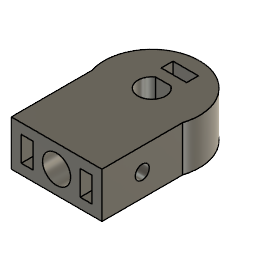
Union_encoder_péndulo (Autodesk Fusion 360 design; units mm, degrees)
Autodesk Fusion 360 part; units mm, degrees
sketch "Sketch1" plane through (0, 0, 0) normal (0, 0, 1) x (1, 0, 0)
  circle A0 centre (0, 0) radius 3.05
  circle A1 centre (0, 0) radius 10.5
  line L0 (-0.015271, 2.53) -> (-0.015271, 6.18)
  line L1 (-0.021322, 3.050767) -> (2.691698, 4.610144)
  line L2 (2.691698, 4.610144) -> (2.697749, 7.739376)
  line L3 (2.697749, 7.739376) -> (-0.009221, 9.309233)
  line L4 (-0.009221, 9.309233) -> (-2.722241, 7.749856)
  line L5 (-2.722241, 7.749856) -> (-2.728292, 4.620624)
  line L6 (-2.728292, 4.620624) -> (-0.021322, 3.050767)
  line L7 (-0.015271, 2.53) -> (1.703408, 2.53)
  line L8 (-0.015271, 2.53) -> (-1.703408, 2.53)
  point P0 (-0.015271, 6.18)
  dimension "d1" = 6.1
  dimension "d3" = 21
  dimension "d14" = 3.65
  dimension "d15" = 2.71
  constraint coincident A0.centre A1.centre
  constraint perpendicular L0 L7
  constraint perpendicular L0 L8
  measures "d1" diameter of A0
  measures "d3" diameter of A1
extrude "Extrude2" add sketch "Sketch1" along normal blind 8 contours L1 L2 L3 L4 L5 L6 | A0 L0 L7 | A0 L0 L8 | A1 picked at (-0.919611, 5.660208) picked at (0.132593, 2.866279) picked at (-0.165511, 2.864986) picked at (-5.003269, 3.445026)
sketch "Sketch3" plane through (0, 0, 8) normal (0, 0, 1) x (-1, 0, 0)
  circle A0 centre (0, 0) radius 10.5
  line L0 (0, 0) -> (0, -2.58)
  line L1 (0, -2.58) -> (0, -6.18)
  line L2 (-2.714531, -4.623256) -> (-2.705446, -7.752481)
  line L3 (-2.705446, -7.752481) -> (0.009086, -9.309225)
  line L4 (0.009086, -9.309225) -> (2.714531, -7.736744)
  line L5 (2.714531, -7.736744) -> (2.705446, -4.607519)
  line L6 (2.705446, -4.607519) -> (-0.009086, -3.050775)
  line L7 (-0.009086, -3.050775) -> (-2.714531, -4.623256)
  line L8 (2.75, -4.88) -> (-2.75, -4.88)
  line L9 (-2.75, -4.88) -> (-2.75, -7.48)
  line L10 (-2.75, -7.48) -> (2.75, -7.48)
  line L11 (2.75, -7.48) -> (2.75, -4.88)
  line L12 (2.75, -4.88) -> (-2.75, -7.48) construction
  line L13 (-2.75, -4.88) -> (2.75, -7.48) construction
  line L14 (1.703408, -2.53) -> (-1.703408, -2.53)
  arc A1 (1.703408, -2.53) -> (-1.703408, -2.53) centre (0, 0) ccw
  point P0 (0, -6.18)
  point P1 (0, -6.18)
  dimension "d18" = 2.58
  dimension "d19" = 3.6
  dimension "d20" = 2.71
  dimension "d36" = 5.5
  dimension "d37" = 2.6
  constraint coincident A0.centre L0.start
  constraint vertical L0
  constraint parallel L0 L1
  constraint coincident P1 P0
  constraint horizontal L8
  constraint perpendicular L8 L9
  constraint parallel L8 L10
  constraint parallel L9 L11
  constraint coincident L12 P1
  constraint coincident L13 P1
  measures "d18" distance of A0.centre L0.end
  measures "d19" distance of L0.end P1
  measures "d20" distance of P1 L7
  measures "d36" distance of L9.end L10.end
  measures "d37" distance of L8.end L9.end
ref_plane "WorkPlane2" through (0, 9.309, 0) normal (0, 1, 0) x (0, 0, 1)
sketch "Sketch4" plane through (0, 9.309, 0) normal (0, 1, 0) x (1, 0, 0)
  line L0 (0, 0) -> (0, -4)
  line L1 (0, -4) -> (-2.71, -4)
  line L2 (-2.71, -4) -> (2.71, -4)
  line L3 (2.71, -4) -> (2.71, -6.6)
  line L4 (2.71, -6.6) -> (-2.71, -6.6)
  line L5 (-2.71, -6.6) -> (-2.71, -4)
  circle A0 centre (0, -4) radius 1.55
  line L6 (-0.007452, -0.87077) -> (-2.713718, -2.441839)
  line L7 (-2.713718, -2.441839) -> (-2.706266, -5.571068)
  line L8 (-2.706266, -5.571068) -> (0.007452, -7.12923)
  line L9 (0.007452, -7.12923) -> (2.713718, -5.558161)
  line L10 (2.713718, -5.558161) -> (2.706266, -2.428932)
  line L11 (2.706266, -2.428932) -> (-0.007452, -0.87077)
  point P0 (0, -4)
  point P1 (0, -4)
  dimension "d25" = 4
  dimension "d26" = 2.71
  dimension "d27" = 5.42
  dimension "d28" = 2.6
  dimension "d38" = 3.1
  dimension "d39" = 2.71
  constraint coincident L0.start origin
  constraint vertical L0
  constraint perpendicular L0 L1
  constraint horizontal L2
  constraint vertical L3
  constraint horizontal L4
  constraint vertical L5
  constraint coincident P1 P0
  measures "d25" distance of L0.start P0
  measures "d26" distance of P1 L1.end
  measures "d27" distance of L1.end L2.end
  measures "d28" distance of L2 L4
  measures "d38" diameter of A0
  measures "d39" distance of P1 L11
extrude "Extrude7" cut sketch "Sketch4" against normal blind 4.5 contours L0 L2 A0 L10 L11 | L0 L1 L2 A0 L6 L7 L11 picked at (1.18142, -2.000013) picked at (-1.186388, -2.002889)
extrude "Extrude8" cut sketch "Sketch4" along normal blind 1.16236 contours L0 L2 A0 | L0 L1 L2 A0 | L1 L2 A0 picked at (0.825118, -3.382324) picked at (-0.825118, -3.382324) picked at (-1.027563, -4.077005)
extrude "Extrude9" cut sketch "Sketch4" against normal blind 7 contours L0 L2 A0 | L0 L1 L2 A0 | L1 L2 A0 picked at (0.825118, -3.382324) picked at (-0.825118, -3.382324) picked at (-1.027563, -4.077005)
extrude "Extrude10" cut sketch "Sketch4" along normal blind 2 contours L0 L2 A0 | L0 L1 L2 A0 | L1 L2 A0 picked at (0.825118, -3.382324) picked at (-0.825118, -3.382324) picked at (-1.027563, -4.077005)
extrude "Extrude11" cut sketch "Sketch3" against normal blind 4 contours L2 L5 L8 L10 picked at (0.002516, -6.613333)
extrude "Extrude12" add sketch "Sketch4" against normal blind 1.8 contours L0 L2 A0 L10 L11 | L0 L1 L2 A0 L6 L7 L11 picked at (1.18142, -2.000013) picked at (-1.186388, -2.002889)
ref_plane "WorkPlane3" through (0, -11, 0) normal (0, 1, 0) x (0, 0, 1)
sketch "Sketch5" plane through (0, -11, 0) normal (0, 1, 0) x (1, 0, 0)
  line L0 (0, 0) -> (10, 0)
  line L1 (10, 0) -> (-10, 0)
  line L2 (-10, 0) -> (-10, -8)
  line L3 (-10, -8) -> (10, -8)
  line L4 (10, -8) -> (10, 0)
  circle A0 centre (0, -4) radius 4
  circle A1 centre (0, -4) radius 3.1
  dimension "d53" = 10
  dimension "d54" = 20
  dimension "d55" = 6.2
  constraint coincident L0.start origin
  constraint horizontal L0
  constraint horizontal L1
  constraint vertical L2
  constraint horizontal L3
  constraint vertical L4
  constraint coincident L0.start A0
  constraint concentric A0 A1
  measures "d53" distance of L0.start L0.end
  measures "d54" distance of L0.end L1.end
  measures "d55" diameter of A1
extrude "Extrude13" cut sketch "Sketch5" along normal blind 5 contours A1 picked at (0.859819, -5.398205)
extrude "Extrude14" add sketch "Sketch5" along normal up to surface contours A0 picked at (-0.275944, -7.682218) end surface at (3.090116, 10.034998, 4)
extrude "Extrude15" add sketch "Sketch5" along normal up to surface contours L1 L2 L3 A0 | L0 L1 L3 L4 A0 picked at (-7.996272, -4.09964) picked at (8, -4) end surface at (-5.243432, -9.097055, 3.949693)
extrude "Extrude16" add 1 faces at (-7.7, -11, 4) along direction (0, -1, 0) blind 10
extrude "Extrude17" add 2 faces at (-0.25937, -17.490376, 8) (-4.991119, 3.5318, 8) along direction (0, 0, 1) blind 1
extrude "Extrude18" add 1 faces at (0, -15.016667, 0) along direction (0, 0, -1) blind 1
sketch "Sketch6" plane through (10, 0, 0) normal (1, 0, 0) x (0, 1, 0)
  line L0 (-3.201562, -1) -> (-3.201562, 9)
  line L1 (-3.201562, 9) -> (-21, 9)
  line L2 (-21, 9) -> (-21, -1)
  line L3 (-21, -1) -> (-3.201562, -1)
  line L4 (-21, -1) -> (-12.100781, -1)
  line L5 (-12.100781, -1) -> (-12.100781, 4) construction
  line L6 (-13.6654, 6.71) -> (-15.23002, 4)
  line L7 (-15.23002, 4) -> (-13.6654, 1.29)
  line L8 (-13.6654, 1.29) -> (-10.536162, 1.29)
  line L9 (-10.536162, 1.29) -> (-8.971543, 4)
  line L10 (-8.971543, 4) -> (-10.536162, 6.71)
  line L11 (-10.536162, 6.71) -> (-13.6654, 6.71)
  circle A0 centre (-12.100781, 4) radius 1.55
  line L12 (-12.100781, 6.71) -> (-12.100781, 1.29)
  point P0 (-12.100781, 4)
  dimension "d68" = 5
  dimension "d69" = 2.71
  dimension "d73" = 3.1
  constraint coincident L2.end L3.start
  constraint perpendicular L4 L5
  measures "d73" diameter of A0
sketch "Sketch7" plane through (0, -21, 0) normal (0, -1, 0) x (1, 0, 0)
  circle A0 centre (0, 4) radius 3.1
  line L0 (-10, 9) -> (-10, -1)
  line L1 (-10, -1) -> (10, -1)
  line L2 (10, -1) -> (10, 9)
  line L3 (10, 9) -> (-10, 9)
  line L4 (10, -1) -> (3, -1)
  line L5 (3, -1) -> (3, 9) construction
  line L6 (3, 9) -> (10, 9)
  line L7 (10, 9) -> (10, -1)
  line L8 (6.5, -1) -> (6.5, 4) construction
  line L9 (5.2, 1.25) -> (7.8, 1.25)
  line L10 (7.8, 1.25) -> (7.8, 6.75)
  line L11 (7.8, 6.75) -> (5.2, 6.75)
  line L12 (5.2, 6.75) -> (5.2, 1.25)
  line L13 (5.2, 1.25) -> (7.8, 6.75) construction
  line L14 (7.8, 1.25) -> (5.2, 6.75) construction
  line L15 (0, 9) -> (0, -1) construction
  line L16 (-5.2, 6.75) -> (-5.2, 1.25)
  line L17 (-7.8, 6.75) -> (-5.2, 6.75)
  line L18 (-7.8, 1.25) -> (-7.8, 6.75)
  line L19 (-5.2, 1.25) -> (-7.8, 1.25)
  point P0 (6.5, 4)
  dimension "d70" = 5
  dimension "d71" = 2.6
  dimension "d72" = 5.5
  constraint horizontal L4
  constraint vertical L5
  constraint horizontal L6
  constraint vertical L7
  constraint coincident L3 L5.end
  constraint coincident L1.end L2.start
  constraint midpoint L4 L8.start
  constraint perpendicular L4 L8
  constraint horizontal L9
  constraint perpendicular L9 L10
  constraint parallel L9 L11
  constraint parallel L10 L12
  constraint coincident L13 P0
  constraint coincident L14 P0
  constraint coincident P0 L8.end
  constraint midpoint L3 L15.start
  constraint midpoint L1 L15.end
  constraint symmetric L9.start L15 L16.end
  constraint symmetric L9.end L15 L18.start
  constraint symmetric L10.end L15 L17.start
  constraint symmetric L11.end L15 L16.start
  measures "d70" distance of L8.start P0
  measures "d71" distance of L10.end L11.end
  measures "d72" distance of L9.end L10.end
extrude "Extrude19" cut sketch "Sketch6" along normal up to surface contours A0 L12 | A0 L12 picked at (-12.616003, 4.038611) picked at (-11.157335, 3.582149) end surface at (3.084595, -16, 4.30866)
extrude "Extrude20" cut sketch "Sketch6" against normal blind 4.8 contours L8 L9 L10 L11 A0 L12 picked at (-10.101514, 2.817336)
extrude "Extrude21" add sketch "Sketch6" against normal blind 2.2 contours L6 L7 L8 L11 A0 L12 | L8 L9 L10 L11 A0 L12 picked at (-14.112847, 2.838333) picked at (-10.101514, 2.817336)
extrude "Extrude22" cut sketch "Sketch7" against normal blind 9 contours L9 L10 L11 L12 picked at (6.933333, 3.083333)
sketch "Sketch8" plane through (-10, 0, 0) normal (-1, 0, 0) x (0, -1, 0)
  line L0 (3.201562, 9) -> (3.201562, -1)
  line L1 (3.201562, -1) -> (21, -1)
  line L2 (21, -1) -> (21, 9)
  line L3 (21, 9) -> (3.201562, 9)
  line L4 (12.100781, -1) -> (12.100781, 4)
  line L5 (13.6654, 1.29) -> (15.23002, 4)
  line L6 (15.23002, 4) -> (13.6654, 6.71)
  line L7 (13.6654, 6.71) -> (10.536162, 6.71)
  line L8 (10.536162, 6.71) -> (8.971543, 4)
  line L9 (8.971543, 4) -> (10.536162, 1.29)
  line L10 (10.536162, 1.29) -> (13.6654, 1.29)
  circle A0 centre (12.100781, 4) radius 1.55
  line L11 (12.100781, 6.71) -> (12.100781, 1.5)
  point P0 (12.100781, 4)
  dimension "d82" = 5
  dimension "d83" = 2.71
  dimension "d84" = 3.1
  constraint perpendicular L1 L4
  constraint perpendicular L10 L11
  measures "d84" diameter of A0
extrude "Extrude23" cut sketch "Sketch8" against normal blind 4.8 contours L4 L7 L8 L9 L10 A0 L11 picked at (10.088715, 5.161667)
extrude "Extrude24" cut sketch "Sketch8" along normal up to surface contours L4 A0 L11 | L4 A0 L11 picked at (12.023776, 2.972437) picked at (13.128855, 3.926471) end surface at (2.147445, -16, 1.764272)
extrude "Extrude25" add sketch "Sketch8" against normal blind 2.2 contours L4 L7 L8 L9 L10 A0 L11 picked at (10.088715, 5.161667)
extrude "Extrude26" cut sketch "Sketch7" against normal blind 9 contours L16 L17 L18 L19 picked at (-6.066667, 4.916667)
sketch "Boceto9" plane through (0, 0, 9) normal (0, 0, 1) x (-1, 0, 0)
  line L0 (2.713786, -7.48) -> (-2.706237, -7.48)
  line L1 (-2.706237, -7.48) -> (-2.713786, -4.88)
  line L2 (-2.713786, -4.88) -> (2.706237, -4.88)
  line L3 (2.706237, -4.88) -> (2.713786, -7.48)
  line L4 (1.703408, -2.53) -> (-1.703408, -2.53)
  arc A0 (1.703408, -2.53) -> (-1.703408, -2.53) centre (0, 0) ccw
  arc A1 (-10, 3.201562) -> (10, 3.201562) centre (0, 0) ccw
  line L5 (10, 3.201562) -> (10, 21)
  line L6 (10, 21) -> (-10, 21)
  line L7 (-10, 21) -> (-10, 3.201562)
  line L8 (-2.796225, -4.88) -> (2.803775, -4.88)
  line L9 (2.803775, -4.88) -> (2.803775, -7.48)
  line L10 (2.803775, -7.48) -> (-2.796225, -7.48)
  line L11 (-2.796225, -7.48) -> (-2.796225, -4.88)
  line L12 (-2.796225, -4.88) -> (2.803775, -7.48) construction
  line L13 (2.803775, -4.88) -> (-2.796225, -7.48) construction
  point P0 (0.003775, -6.18)
  dimension "d93" = 5.6
  constraint horizontal L8
  constraint perpendicular L8 L9
  constraint parallel L8 L10
  constraint parallel L9 L11
extrude "Extruir27" cut sketch "Boceto9" against normal blind 6.5 contours L3 L8 L9 L10 | L1 L8 L10 L11 picked at (2.741266, -5.746667) picked at (-2.738749, -6.613333)
equation "d26 = ( 5.42 / 2 ) * 1 mm"
